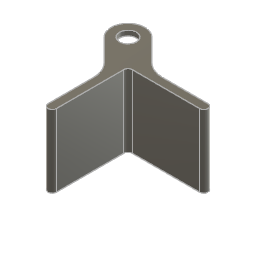
Culture Retainer v2 (Autodesk Fusion 360 design; units mm, degrees)
Autodesk Fusion 360 part; units mm, degrees
note: some values were not read from the file. Set by a fixed rule: which sketch regions a step uses.
sketch "Sketch1" plane through (0, 0, 0) normal (0, 1, 0) x (1, 0, 0)
  circle A0 centre (0, 0) radius 2
  line L0 (0, 0) -> (4.2, -4.2) construction
  line L1 (4.2, -4.2) -> (24.2, -4.2)
  line L2 (24.2, -4.2) -> (24.2, -6.2)
  line L3 (24.2, -6.2) -> (4.2, -6.2)
  line L4 (4.2, -6.2) -> (4.2, -4.2)
  line L5 (4.2, -4.2) -> (6.2, -4.2)
  line L6 (6.2, -4.2) -> (6.2, -24.2)
  line L7 (6.2, -24.2) -> (4.2, -24.2)
  line L8 (4.2, -24.2) -> (4.2, -4.2)
  line L9 (4.2, -9.8569) -> (-5.6569, 0)
  line L10 (-5.6569, 0) -> (0, 5.6569)
  line L11 (0, 5.6569) -> (9.8569, -4.2)
  line L12 (0, 0) -> (-2.8284, 2.8284)
  dimension "d1" = 4
  dimension "d2" = 4.2
  dimension "d3" = 4.2
  dimension "d4" = 2
  dimension "d5" = 20
  dimension "d6" = 135
  dimension "d7" = 4
  dimension "d8" = 8
  constraint coincident A0.centre L0.start
  constraint horizontal L1
  constraint vertical L2
  constraint horizontal L3
  constraint vertical L4
  constraint horizontal L5
  constraint vertical L6
  constraint horizontal L7
  constraint vertical L8
  constraint equal L2 L7
  constraint equal L1 L6
  constraint coincident L8 L9.start
  constraint perpendicular L9 L10
  constraint coincident L1 L11.end
  constraint perpendicular L10 L11
  constraint perpendicular L10 L12
  constraint midpoint L10 L12.end
  measures "d1" diameter of A0
  measures "d2" horizontal distance of A0.centre L0.end
  measures "d3" vertical distance of A0.centre L0.end
  measures "d4" distance of L1.end L2.end
  measures "d5" distance of L0.end L1.end
  measures "d6" angle of L1 L11
  measures "d7" distance of A0.centre L12.end
  measures "d8" distance of L9.end L10.end
extrude "Extrude1" add sketch "Sketch1" along normal blind 1.2
fillet "Fillet1" radius 1 5 edges at (6.2, 0.6, 6.2) (6.2, 0.6, 24.2) (4.2, 0.6, 24.2) (24.2, 0.6, 6.2) (24.2, 0.6, 4.2)
fillet "Fillet2" radius 4 2 edges at (-5.6569, 0.6, 0) (0, 0.6, -5.6569)
fillet "Fillet3" radius 6 2 edges at (4.2, 0.6, 9.8569) (9.8569, 0.6, 4.2)
sketch "Sketch2" plane through (0, 0, 0) normal (0, -1, 0) x (1, 0, 0)
  arc A0 (-2.8284, 2.8284) -> (2.8284, -2.8284) centre (0, 0) ccw
  line L0 (2.8284, -2.8284) -> (8.0995, 2.4426)
  arc A1 (12.3421, 4.2) -> (8.0995, 2.4426) centre (12.3421, -1.8) ccw
  line L1 (12.3421, 4.2) -> (23.2, 4.2)
  arc A2 (23.2, 4.2) -> (23.2, 6.2) centre (23.2, 5.2) ccw
  line L2 (23.2, 6.2) -> (7.2, 6.2)
  arc A3 (6.2, 7.2) -> (7.2, 6.2) centre (7.2, 7.2) ccw
  line L3 (6.2, 7.2) -> (6.2, 23.2)
  arc A4 (6.2, 23.2) -> (4.2, 23.2) centre (5.2, 23.2) ccw
  line L4 (4.2, 23.2) -> (4.2, 12.3421)
  arc A5 (2.4426, 8.0995) -> (4.2, 12.3421) centre (-1.8, 12.3421) ccw
  line L5 (2.4426, 8.0995) -> (-2.8284, 2.8284)
  circle A6 centre (0, 0) radius 2
  line L6 (4.2, 23.2) -> (4.2, 4.2)
  line L7 (4.2, 4.2) -> (23.2, 4.2)
  constraint coincident A4.end L4.start
  constraint coincident L1.end A2.start
  constraint perpendicular L6 L7
  constraint equal L6 L7
extrude "Extrude2" add sketch "Sketch2" along normal blind 16 contours L1 A2 L2 A3 L3 A4 L4 L6 L7
fillet "Fillet4" radius 2 1 edges at (4.2, -8, 4.2)
equation "d6 = 180 deg - 45 deg"
